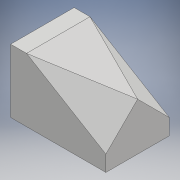
# Autodesk Inventor part: 16
Saved by Autodesk Inventor 2017 (Build 210142000, 142)
## iProperties
Part Number: 16
Material: 一般
Document SubType Name: Modeling
Designer: Brian
Density: 1 g/cm^3
Appearance: 預設
Author: Brian
Autodesk Inventor part; units mm, degrees
ref_plane "YZ Plane" through (0, 0, 0) normal (1, 0, 0) x (0, 1, 0)
ref_plane "XZ Plane" through (0, 0, 0) normal (0, 1, 0) x (-1, 0, 0)
sketch "草圖1" plane through (0, 0, 0) normal (0, 1, 0) x (-1, 0, 0)
  line L0 (0, 0) -> (-60, 0)
  line L1 (-60, 0) -> (-60, -40)
  line L2 (-60, -40) -> (0, -40)
  line L3 (0, -40) -> (0, 0)
  dimension "d0" = 60
  dimension "d1" = 40
  constraints: 8 end point, 2 parallel, 1 horizontal, 1 perpendicular
  measures "d0" distance of L1.end L2.end
  measures "d1" distance of L2.end L0.start
extrude "擠出1" add sketch "草圖1" along normal mid plane 40
sketch "草圖2" plane through (0, 20, 0) normal (0, 1, 0) x (1, 0, 0)
  line L0 (0, 0) -> (60, 0) projected
  line L1 (10, 0) -> (60, 10)
  line L2 (60, 0) -> (60, 40) projected
  dimension "d4" = 10
  dimension "d5" = 30
  constraints: 2 end point, 2 point on line
  measures "d4" distance of L0.start L1.start
  measures "d5" distance of L2.end L1.end
extrude "擠出2" cut sketch "草圖2" against normal blind 40
sketch "草圖3" plane through (60, -20, -40) normal (1, 0, 0) x (0, 0, -1)
  line L0 (-30, 20) -> (-10, 40)
  line L1 (0, 40) -> (-40, 40) projected
  line L2 (-30, 40) -> (-30, 0) projected
  point P0 (-40, 20)
  dimension "d8" = 20
  dimension "d9" = 20
  constraints: 2 end point, 1 midpoint, 1 point on line
  measures "d8" horizontal distance of L0.start L0.end
  measures "d9" horizontal distance of L0.start L0.end
ref_plane "工作平面1" through (10, 20, 0) normal (-0.3906, -0.6509, -0.6509) x (0.8575, 0, -0.5145)
sketch "草圖4" plane through (10, 20, 0) normal (-0.3906, -0.6509, -0.6509) x (0.8575, 0, -0.5145)
  line L0 (-15.1543, -12.3218) -> (93.717, -12.3218)
  line L1 (93.717, -12.3218) -> (93.717, 28.8166)
  line L2 (93.717, 28.8166) -> (-15.1543, 28.8166)
  line L3 (-15.1543, 28.8166) -> (-15.1543, -12.3218)
  point P0 (-8.5749, 11.8334)
  constraints: 8 end point, 2 parallel, 1 horizontal, 1 perpendicular
extrude "擠出3" cut sketch "草圖4" against normal blind 40
mirror "鏡射1" about plane through (0, 0, 0) normal (0, 1, 0) of "擠出3"
